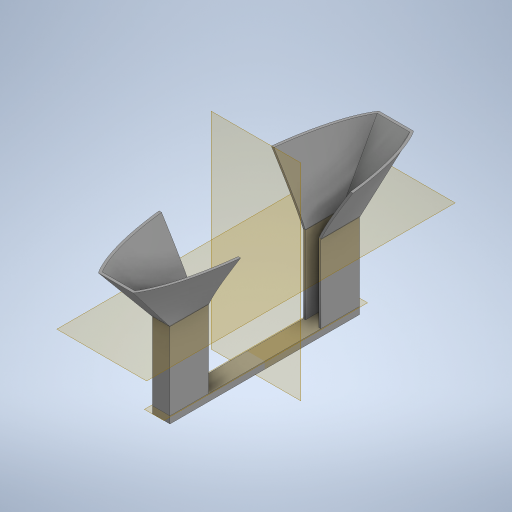
# Autodesk Inventor part: Landing Docks Third Iteration 2
Saved by Autodesk Inventor 2023 (Build 270158000, 158)
## iProperties
Created: 2023-02-15
Part Number: Landing Docks Third Iteration 2
Material: PLA 33 Plastic
Document SubType Name: Modeling
Designer: mihal
Density: 0.4135 g/cm^3
Appearance: Generic
Mass: 93.94 g
Surface Area: 1382.15 cm^2
Volume: 227.183 cm^3
Author: mihal
Autodesk Inventor part; units mm, degrees
ref_plane "YZ Plane" through (0, 0, 0) normal (1, 0, 0) x (0, 1, 0)
ref_plane "XZ Plane" through (0, 0, 0) normal (0, 1, 0) x (-1, 0, 0)
ref_plane "XY Plane" through (0, 0, 0) normal (0, 0, 1) x (1, 0, 0)
sketch "Sketch29" plane through (0, 0, 0) normal (0, 1, 0) x (-1, 0, 0)
  line L0 (-12.5, 135) -> (12.5, 135)
  line L1 (12.5, 135) -> (12.5, -135)
  line L2 (12.5, -135) -> (-12.5, -135)
  line L3 (-12.5, -135) -> (-12.5, 135)
  line L4 (-12.5, 135) -> (12.5, -135) construction
  line L5 (12.5, 135) -> (-12.5, -135) construction
  point P0 (0, 0)
  dimension "d212" = 25
  dimension "d213" = 270
  constraints: 12 end point, 2 midpoint, 2 parallel, 1 horizontal, 1 perpendicular
  measures "d212" distance of L1.end L2.end
  measures "d213" distance of L2.end L0.start
extrude "Extrusion23" add sketch "Sketch29" along normal blind 120
ref_plane "Work Plane6" through (0, 220, 0) normal (0, 1, 0) x (1, 0, 0)
sketch "Sketch31" plane through (0, 0, 0) normal (1, 0, 0) x (0, 1, 0)
  line L0 (3, -132) -> (3, 132) projected
  line L1 (266.8358, 80) -> (3, 80)
  line L2 (3, 80) -> (3, -80)
  line L3 (3, -80) -> (266.8358, -80)
  line L4 (266.8358, -80) -> (266.8358, 80)
  line L5 (266.8358, 80) -> (3, -80) construction
  line L6 (3, 80) -> (266.8358, -80) construction
  line L7 (-53.3672, 0) -> (320.203, 0) projected
  point P0 (0, 0)
  point P1 (134.9179, 0)
  point P2 (3, 80)
  dimension "d226" = 160
  constraints: 12 end point, 2 midpoint, 2 parallel, 2 point on line, 1 horizontal, 1 perpendicular
  measures "d226" distance of L3.end L1.start
ref_plane "Work Plane8" through (0, 200, 0) normal (0, 1, 0) x (1, 0, 0)
sketch "Sketch30" plane through (0, 200, 0) normal (0, 1, 0) x (1, 0, 0)
  line L0 (-24.7631, -199.6997) -> (24.7631, -199.6997)
  line L1 (-24.7631, 199.6997) -> (24.7631, 199.6997)
  ellipse E0 centre (0, 0) end of major axis (0, 217.5) minor radius 62.5 (24.7631, -199.6997) -> (24.7631, 199.6997) ccw
  ellipse E1 centre (0, 0) end of major axis (0, 217.5) minor radius 62.5 (-24.7631, 199.6997) -> (-24.7631, -199.6997) ccw
  constraints: 4 end point, 2 horizontal, 1 coincident, 8 other
loft "Loft9" add profiles "Sketch30" section 2 edges at (0, 120, -135) (-12.5, 120, 0) (0, 120, 135) (12.5, 120, 0)
shell "Shell3" thickness 3 removed faces 1 at (-20.7097, 200, -7.8867)
sketch "Sketch41" plane through (12.5, 0, 135) normal (1, 0, 0) x (0, 0, -1)
  line L0 (0, 0) -> (270, 0) projected
  line L1 (270, 0) -> (270, 120) projected
  line L2 (0, 120) -> (270, 120) projected
  line L3 (0, 0) -> (0, 120) projected
  line L4 (270, 120) -> (0, 120) projected
  line L5 (135, 120) -> (135, 200)
  line L6 (334.6997, 200) -> (-64.6997, 200) projected
  line L7 (55, 310) -> (215, 310)
  line L8 (215, 310) -> (215, 10)
  line L9 (215, 10) -> (55, 10)
  line L10 (55, 10) -> (55, 310)
  line L11 (55, 310) -> (215, 10) construction
  line L12 (215, 310) -> (55, 10) construction
  point P0 (135, 0)
  point P1 (135, 160)
  dimension "d292" = 160
  dimension "d293" = 10
  constraints: 14 end point, 5 midpoint, 2 parallel, 1 horizontal, 1 perpendicular
  measures "d292" distance of L8.end L9.end
  measures "d293" distance between parallel lines of L0 L9
extrude "Extrusion33" cut sketch "Sketch41" along normal blind 80 and the other way blind 80 contours L10 L6 L5 L2 | L2 L8 L9 L10 | L2 L5 L6 L8 | L10 L7 L8 L6
sketch "Sketch42" plane through (0, 0, 0) normal (0, -1, 0) x (1, 0, 0)
  line L0 (12.5, -135) -> (-12.5, -135) projected
  line L1 (12.5, 135) -> (12.5, -135) projected
  line L2 (-12.5, 135) -> (12.5, 135) projected
  line L3 (-12.5, -135) -> (-12.5, 135) projected
  circle A0 centre (0, 0) radius 9
  circle A1 centre (0, -60) radius 9
  circle A2 centre (0, 60) radius 9
  dimension "d298" = 18
  dimension "d299" = 18
  dimension "d300" = 18
  dimension "d301" = 60
  dimension "d302" = 60
  constraints: 3 centre point, 1 coincident
  measures "d298" diameter of A0
  measures "d299" diameter of A1
  measures "d300" diameter of A2
  measures "d301" distance of point (0, 0) A2.centre
  measures "d302" distance of point (0, 0) A1.centre
sketch "Sketch43" plane through (-9.5, 3, -132) normal (0, 1, 0) x (1, 0, 0)
  line L0 (19, 0) -> (0, 0) projected
  line L1 (0, 0) -> (0, -264) projected
  line L2 (0, -264) -> (19, -264) projected
  line L3 (19, -264) -> (19, 0) projected
  point P0 (9.5, -132)
extrude "Extrusion34" add sketch "Sketch43" along normal up to surface (7 mm away)
extrude "Extrusion35" cut sketch "Sketch42" against normal blind 7 contours A0 | A1 | A2
ref_plane "Work Plane10" through (0, 121.0613, 132) normal (0, 1, 0) x (1, 0, 0)
ref_plane "Work Plane11" through (12.5, 10, 80) normal (0, 1, 0) x (1, 0, 0)
split body "Split1" result two bodies by plane through (0, 121.0613, 132) normal (0, 1, 0) first body at (-13.371, 124.0974, -105.3291) (13.371, 124.0974, 105.3291)
split body "Split2" result two bodies by plane through (12.5, 10, 80) normal (0, 1, 0) bodies 3 first body at (-12, 46.6667, -116.6667) (-12, 46.6667, 98.3333)
ref_plane "Work Plane12" through (-12.9774, 121.0613, 0) normal (0, 0, 1) x (1, 0, 0)
split body "Split3" result two bodies by plane through (-12.9774, 121.0613, 0) normal (0, 0, 1) bodies 4 first body at (-12, 46.6667, 98.3333)
split body "Split4" result two bodies by plane through (-12.9774, 121.0613, 0) normal (0, 0, 1) bodies 2 first body at (13.371, 124.0974, 105.3291)
body "Solid6"
body "Solid7"
body "Solid8"
body "Solid9"
body "Solid10"
